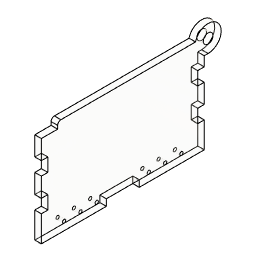
right_and_left_plates (Autodesk Fusion 360 design; units mm, degrees)
Autodesk Fusion 360 part; units mm, degrees
note: some values were not read from the file. Set by a fixed rule: which sketch regions a step uses.
sketch "Esquisse1" plane through (0, 0, 0) normal (1, 0, 0) x (0, 1, 0)
  line L0 (0, 0) -> (-250, 0) construction
  line L1 (-250, 0) -> (-250, 150) construction
  line L2 (-220, 150) -> (0, 150) construction
  line L3 (0, 150) -> (0, 0) construction
  line L4 (0, 0) -> (0, 39.75)
  line L5 (-10, 39.75) -> (0, 39.75)
  line L6 (-10, 39.75) -> (-10, 60.25)
  line L7 (-10, 60.25) -> (0, 60.25)
  line L8 (0, 60.25) -> (0, 89.75)
  line L9 (-10, 89.75) -> (-10, 110.25)
  line L10 (-10, 110.25) -> (0, 110.25)
  line L11 (-10, 89.75) -> (0, 89.75)
  line L12 (0, 110.25) -> (0, 125)
  line L13 (-13.3649, 150) -> (-250, 150) construction
  line L14 (11, 150) -> (1, 150) construction
  line L15 (1, 150) -> (1, 140) construction
  line L16 (1, 140) -> (11, 140) construction
  line L17 (11, 140) -> (11, 150) construction
  line L18 (11, 150) -> (1, 140) construction
  line L19 (1, 150) -> (11, 140) construction
  arc A0 (6, 125) -> (-13.3649, 150) centre (6, 145) ccw
  line L20 (-13.3649, 150) -> (-220, 150)
  line L21 (-250, 140) -> (-250, 110.5)
  line L22 (-250, 110.5) -> (-240, 110.5)
  line L23 (-240, 110.5) -> (-240, 90)
  line L24 (-240, 90) -> (-250, 90)
  line L25 (-250, 90) -> (-250, 60.5)
  line L26 (-250, 60.5) -> (-240, 60.5)
  line L27 (-240, 60.5) -> (-240, 40)
  line L28 (-240, 40) -> (-250, 40)
  line L29 (-250, 40) -> (-250, 0)
  line L30 (-250, 0) -> (-150.25, 0)
  line L31 (-150.25, 0) -> (-150.25, 10)
  line L32 (-150.25, 10) -> (-99.75, 10)
  line L33 (-99.75, 10) -> (-99.75, 0)
  line L34 (-99.75, 0) -> (0, 0)
  line L35 (-125, 150) -> (-125, 10) construction
  line L36 (-250, 75) -> (0, 75) construction
  circle A1 centre (6, 145) radius 7.5
  circle A2 centre (6, 145) radius 7.0711 construction
  line L37 (-125, 150) -> (-125, 0) construction
  line L38 (-225, 145) -> (-225, 140)
  line L39 (-225, 140) -> (-250, 140)
  line L40 (0, 140) -> (-250, 140) construction
  line L41 (0, 125) -> (6, 125)
  arc A3 (6, 125) -> (0, 125.9212) centre (6, 145) ccw construction
  arc A4 (0, 125.9212) -> (6, 125) centre (6, 145) ccw construction
  arc A5 (-220, 150) -> (-225, 145) centre (-220, 145) ccw
  point P0 (6, 145)
  point P1 (-10, 100)
  point P2 (-10, 50)
  dimension "d1" = 250
  dimension "d2" = 150
  dimension "d4" = 20.5
  dimension "d7" = 10
  dimension "d8" = 40
  dimension "d11" = 10
  dimension "d12" = 10
  dimension "d13" = 40
  dimension "d29" = 50.5
  dimension "d30" = 10
  dimension "d36" = 140
  dimension "d37" = 10
  dimension "d38" = 1
  dimension "d40" = 5
  dimension "d41" = 50
  dimension "d42" = 15
  dimension "d43" = 25
  constraint horizontal L0
  constraint vertical L1
  constraint horizontal L2
  constraint vertical L3
  constraint coincident L0.start L3.end
  constraint coincident L3 L4.end
  constraint perpendicular L3 L5
  constraint perpendicular L5 L6
  constraint coincident L3 L7.end
  constraint perpendicular L3 L7
  constraint coincident L3 L8.end
  constraint perpendicular L7 L9
  constraint coincident L3 L10.end
  constraint perpendicular L3 L10
  constraint perpendicular L3 L11
  constraint coincident L3 A3.end
  constraint equal L7 L11
  constraint coincident L13.start A3
  constraint coincident L2 L13.start
  constraint horizontal L14
  constraint perpendicular L14 L15
  constraint parallel L14 L16
  constraint parallel L15 L17
  constraint coincident L18 P0
  constraint coincident L19 P0
  constraint coincident P0 A0.centre
  constraint equal A0 A3
  constraint coincident L1 L21.end
  constraint perpendicular L21 L22
  constraint perpendicular L22 L23
  constraint coincident L1 L24.end
  constraint perpendicular L1 L24
  constraint coincident L1 L25.end
  constraint perpendicular L1 L26
  constraint perpendicular L26 L27
  constraint coincident L1 L28.end
  constraint perpendicular L1 L28
  constraint perpendicular L0 L29
  constraint coincident L0 L30.end
  constraint perpendicular L30 L31
  constraint perpendicular L31 L32
  constraint coincident L0 L33.end
  constraint perpendicular L0 L33
  constraint equal L10 L22
  constraint equal L9 L23
  constraint equal L8 L25
  constraint equal L6 L27
  constraint equal L24 L26
  constraint midpoint L32 L35.end
  constraint vertical L35
  constraint midpoint L1 L36.start
  constraint midpoint L8 L36.end
  constraint concentric A0 A1
  constraint coincident L14.start A2
  constraint midpoint L0 L37.end
  constraint coincident L35 L37.start
  constraint coincident L13 L35.start
  constraint perpendicular L20 L38
  constraint perpendicular L38 L39
  constraint coincident L3 L40.start
  constraint coincident L1 L21.start
  constraint horizontal L40
  constraint coincident L3 L12.end
  constraint tangent A0 L41
  constraint horizontal L41
  constraint concentric A0 A4
  constraint coincident L2 L35.start
  constraint coincident L1.end L2
  constraint tangent L38 A5
  constraint tangent L2 A5
  constraint vertical L37
  constraint equal L6 L9
  constraint symmetric L7.end L8.end L36
  constraint midpoint L9 P1
  constraint midpoint L6 P2
  constraint coincident L39 L21.start
  constraint vertical L21
  measures "d1" distance of L0.start L0.end
  measures "d2" distance of L0.start L2.end
  measures "d4" distance of L5 L7
  measures "d7" distance of L3 L6
  measures "d8" diameter of A3
  measures "d11" distance of L15.end L16.end
  measures "d12" distance of L14.end L15.end
  measures "d13" distance of L0 L27.end
  measures "d29" distance of L31.end L32.end
  measures "d30" distance of L0 L32
  measures "d36" distance of L0 L40
  measures "d37" distance of L2 L16
  measures "d38" distance of L3 L15
  measures "d40" radius of A5
  measures "d41" distance of P1 P2
  measures "d42" diameter of A1
  measures "d43" distance of L38.end L21.start
extrude "Extrusion1" add sketch "Esquisse1" along normal blind 10
sketch "Esquisse2" plane through (10, 0, 0) normal (1, 0, 0) x (0, 1, 0)
  circle A0 centre (6, 145) radius 7.5
  line L0 (-250, 140) -> (-250, 110.5)
  line L1 (-250, 110.5) -> (-240, 110.5)
  line L2 (-240, 110.5) -> (-240, 90)
  line L3 (-240, 90) -> (-250, 90)
  line L4 (-250, 90) -> (-250, 60.5)
  line L5 (-250, 60.5) -> (-240, 60.5)
  line L6 (-240, 60.5) -> (-240, 40)
  line L7 (-240, 40) -> (-250, 40)
  line L8 (-250, 40) -> (-250, 0)
  line L9 (-250, 0) -> (-150.25, 0)
  line L10 (-150.25, 0) -> (-150.25, 10)
  line L11 (-150.25, 10) -> (-99.75, 10)
  line L12 (-99.75, 10) -> (-99.75, 0)
  line L13 (-99.75, 0) -> (0, 0)
  line L14 (0, 0) -> (0, 39.75)
  line L15 (0, 39.75) -> (-10, 39.75)
  line L16 (-10, 39.75) -> (-10, 60.25)
  line L17 (-10, 60.25) -> (0, 60.25)
  line L18 (0, 60.25) -> (0, 89.75)
  line L19 (0, 89.75) -> (-10, 89.75)
  line L20 (-10, 89.75) -> (-10, 110.25)
  line L21 (-10, 110.25) -> (0, 110.25)
  line L22 (0, 110.25) -> (0, 125)
  arc A1 (6, 125) -> (-13.3649, 150) centre (6, 145) ccw
  line L23 (-13.3649, 150) -> (-220, 150)
  line L24 (-250, 12.7) -> (0, 12.7) construction
  circle A2 centre (-215, 12.7) radius 2.5
  circle A3 centre (-190, 12.7) radius 2.5
  circle A4 centre (-165, 12.7) radius 2.5
  line L25 (-250, 10.2) -> (0, 10.2) construction
  line L26 (-125, 140) -> (-125, 10)
  circle A5 centre (-35, 12.7) radius 2.5
  circle A6 centre (-85, 12.7) radius 2.5
  circle A7 centre (-60, 12.7) radius 2.5
  line L27 (-225, 145) -> (-225, 140)
  line L28 (-225, 140) -> (-250, 140)
  line L29 (0, 125) -> (6, 125)
  arc A8 (-220, 150) -> (-225, 145) centre (-220, 145) ccw
  point P0 (0, 12.7)
  point P1 (0, 10.2)
  dimension "d22" = 5
  dimension "d24" = 0.2
  dimension "d25" = 25
  dimension "d26" = 25
  dimension "d27" = 35
  constraint coincident L8 L24.start
  constraint coincident L14 P0
  constraint perpendicular L14 L24
  constraint coincident L24 A2.centre
  constraint coincident L24 A3.centre
  constraint coincident L24 A4.centre
  constraint equal A3 A4
  constraint equal A2 A3
  constraint coincident L8 L25.start
  constraint coincident L14 P1
  constraint perpendicular L14 L25
  constraint tangent A2 L25
  constraint midpoint L11 L26.end
  constraint symmetric L24.start L26 P0
  constraint symmetric A2 L26 A5
  constraint symmetric A3 L26 A7
  constraint symmetric A4 L26 A6
  constraint symmetric L25.start L26 P1
  measures "d22" diameter of A2
  measures "d24" distance of L11 L25
  measures "d25" distance of A2.centre A3.centre
  measures "d26" distance of A3.centre A4.centre
  measures "d27" distance of L8 A2.centre
extrude "Extrusion2" cut sketch "Esquisse2" against normal through all contours A2 | A3 | A4 | A5 | A6 | A7
